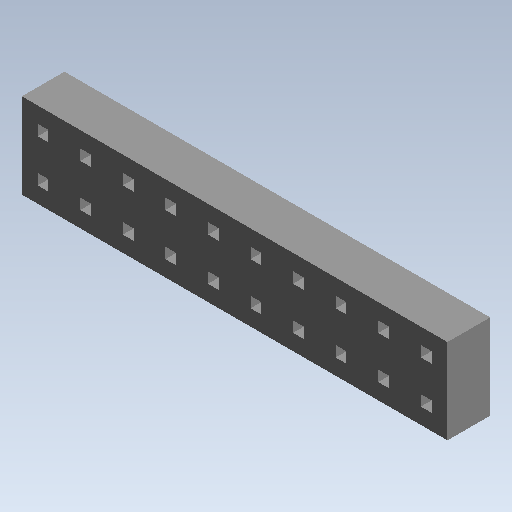
# Autodesk Inventor part: TB2TW-10-11-T-D-250-080
Saved by Autodesk Inventor 2021 (Build 250183000, 183)
## iProperties
Part Number: TB2TW-10-11-T-D-250-080
Material: Generic
Catalog Web Link: www.cadenas.de
Description: TW-TH Series Top Body-TW-TH Series
Vendor: SAMTEC
Document SubType Name: Modeling
Designer: partserver
Manufacturer: SAMTEC
Mass: 0.150089 g
Surface Area: 3.27452 cm^2
Volume: 0.150089 cm^3
Density: 1 g/cm^3
Appearance: PSOLRGB-175-175-175
Category: PARTsolutions
Company: SAMTEC
PSOL_IDENT_0: {$CADENAS_DATA\23d-libs\samtec\modelling\tw\parts\tw-th_top_body.prj},257 {VTYP=3D},{NB=TB2TW-10-11-
PSOL_IDENT_1: T-D-250-080},{LINA=TB2TW-10-11-T-D-250-080},{NN=TW-TH Series Top Body},{DATE=29.08.2019 09:17:19},{G
PSOL_IDENT_2: EOMDATE=10.06.2019 09:16:53},{VERSION=},{LINEID=10},{WBVAR=PINS,LEADST,PLOPT,ROWOPT,STACKERH,TAILL,P
PSOL_IDENT_3: OLARIZE},{WBNUMERIC=STACKERH}  {NB=TB2TW-10-11-T-D-250-080},{LINA=TB2TW-10-11-T-D-250-080},{KT=DUMMY
PSOL_IDENT_4: },{PN=TW-10-11-T-D-250-080},{SERIES=TW-TH},{PINS=10},{LEADST=11},{LEADSTALG=},{PLOPT=T},{PLOPTALG= '
PSOL_IDENT_5: -L','10micro\" (0,25 microm) Gold on contact, Matte Tin on tail','-S','30micro\" (0,76 microm) Gold
PSOL_IDENT_6: on contact, Matte Tin on tail' },{ROWOPT=D},{ROWOPTALG= '5','5:Five Row','6','6:Six Row','D','D:Doub
PSOL_IDENT_7: le Row','Q','Q:Quad Row','S','S:Single row','T','T:Triple Row' },{STACKERH=250},{STACKERHALG=[120:39
PSOL_IDENT_8: 7/5]},{TAILL=080},{TAILLALG='000','005','010','015','020','025','030','035','040','045','050','055','
PSOL_IDENT_9: 060','065','070','075','080','085','090','095','100','105','110','115','120','125','130','135','140'
PSOL_IDENT_10: ,'145'},{ALIGNMENTALG=x},{POLARIZE=Not Selected},{POLARIZEALG='001','002','003','004','005','006','0
PSOL_IDENT_11: 07','008','009','010','011','012','013','014','015','016','017','018','019','020'},{POLARIZEPN=},{KO
PSOL_IDENT_12: PTALG= '','Not Selected','-P','P:Plastic Pick and Place Pad' },{TROPTALG= '','Not Selected','-TR','T
PSOL_IDENT_13: R:Tape and Reel' },{IMAT=Black Liquid Crystal Polymer},{TM=Phosphor Bronze},{PLAT=Au or Sn over 50mi
PSOL_IDENT_14: cro\" (1,27 microm) Ni},{CR=5.2 A per pin (1 pin powered per row)},{OTEMP=-55°C to +125°C},{ROHSC=Ye
PSOL_IDENT_15: s},{L=0.7874},{W=0.1574},{OAL=0.397},{STACKERHMAX=397},{POLMAX='001','002','003','004','005','006','
PSOL_IDENT_16: 007','008','009','010','011','012','013','014','015','016','017','018','019','020','021','022','023'
PSOL_IDENT_17: ,'024','025','026','027','028','029','030','031','032','033','034','035','036','037','038','039','04
PSOL_IDENT_18: 0','041','042','043','044','045','046','047','048','049','050','051','052','053','054','055','056','
PSOL_IDENT_19: 057','058','059','060','061','062','063','064','065','066','067','068','069','070','071','072','073'
PSOL_IDENT_20: ,'074','075','076','077','078','079','080','081','082','083','084','085','086','087','088','089','09
PSOL_IDENT_21: 0','091','092','093','094','095','096','097','098','099','100','101','102','103','104','105','106','
PSOL_IDENT_22: 107','108','109','110','111','112','113','114','115','116','117','118','119','120','121','122','123'
PSOL_IDENT_23: ,'124','125','126','127','128','129','130','131','132','133','134','135','136','137','138','139','14
PSOL_IDENT_24: 0','141','142','143','144','145','146','147','148','149','150','151','152','153','154','155','156','
PSOL_IDENT_25: 157','158','159','160','161','162','163','164','165','166','167','168','169','170','171','172','173'
PSOL_IDENT_26: ,'174','175','176','177','178','179','180','181','182','183','184','185','186','187','188','189','19
PSOL_IDENT_27: 0','191','192','193','194','195','196','197','198','199','200','201','202','203','204','205','206','
PSOL_IDENT_28: 207','208','209','210','211','212','213','214','215','216','217','218','219','220','221','222','223'
PSOL_IDENT_29: ,'224','225','226','227','228','229','230','231','232','233','234','235','236','237','238','239','24
PSOL_IDENT_30: 0','241','242','243','244','245','246','247','248','249','250','251','252','253','254','255','256','
PSOL_IDENT_31: 257','258','259','260','261','262','263','264','265','266','267','268','269','270','271','272','273'
PSOL_IDENT_32: ,'274','275','276','277','278','279','280','281','282','283','284','285','286','287','288','289','29
PSOL_IDENT_33: 0','291','292','293','294','295','296','297','298','299','300'},{TEST2='001','002','003','004','005'
PSOL_IDENT_34: ,'006','007','008','009','010','011','012','013','014','015','016','017','018','019','020'},{TRUNC=2
PSOL_IDENT_35: 0},{MIN=0.147},{PINSNUM=10},{POLLR=0},{TAILLMAX=147},{TAILLRANGE='000','005','010','015','020','025'
PSOL_IDENT_36: ,'030','035','040','045','050','055','060','065','070','075','080','085','090','095','100','105','11
PSOL_IDENT_37: 0','115','120','125','130','135','140','145','150','155','160','165','170','175','180','185','190','
PSOL_IDENT_38: 195','200','205','210','215','220','225','230','235','240','245','250','255','260','265','270','275'
PSOL_IDENT_39: ,'280','285','290','295','300','305','310','315','320','325','330','335','340','345','350','355','36
PSOL_IDENT_40: 0','365','370','375','380','385','390','395','400','405','410','415','420','425','430','435','440','
PSOL_IDENT_41: 445','450','455','460','465','470','475','480','485','490','495','500','505','510','515','520','525'
PSOL_IDENT_42: ,'530','535','540','545','550','555','560','565','570','575','580','585','590','595','600','605','61
PSOL_IDENT_43: 0','615','620','625','630','635','640','645','650','655','660','665','670','675','680','685','690','
PSOL_IDENT_44: 695','700','705','710','715','720','725','730','735','740','745','750','755','760','765','770','775'
PSOL_IDENT_45: ,'780','785','790','795','800','805','810','815','820','825','830','835','840','845','850','855','86
PSOL_IDENT_46: 0','865','870','875','880','885','890','895','900','905','910','915','920','925','930','935','940','
PSOL_IDENT_47: 945','950','955','960','965','970','975','980','985','990','995'},{TAILLTRUNC=30},{TAILLNUM=0.08},{R
PSOL_IDENT_48: OWNO=2},{POLPLANEPOS=0},{POLPINPOS=0}
NB: TB2TW-10-11-T-D-250-080
NN: TW-TH Series Top Body
NT: TW-TH Series
NBSYN: TB2$PN.
LINA: TB2TW-10-11-T-D-250-080
CATALOG: Samtec
SERIES: TW-TH
PINS: 10
LEADST: 11
PLOPT: -T: Matte Tin Contact and Tail
ROWOPT: D:Double Row
STACKERH: 250
TAILL: 080
POLARIZE: Not Selected
IMAT: Black Liquid Crystal Polymer
TM: Phosphor Bronze
PLAT: Au or Sn over 50micro" (1,27 microm) Ni
CR: 5.2 A per pin (1 pin powered per row)
OTEMP: -55°C to +125°C
ROHSC: Yes
POLMAX: '001','002','003','004','005','006','007','008','009','010','011','012','013','014','015','016','017','018','019','020','021','022','023','024','025','026','027','028','029','030','031','032','033','034','035','036','037','038','039','040','041','042','043','044','045','046','047','048','049','050','051','052','053','054','055','056','057','058','059','060','061','062','063','064','065','066','067','068','069','070','071','072','073','074','075','076','077','078','079','080','081','082','083','084','085','086','087','088','089','090','091','092','093','094','095','096','097','098','099','100','101','102','103','104','105','106','107','108','109','110','111','112','113','114','115','116','117','118','119','120','121','122','123','124','125','126','127','128','129','130','131','132','133','134','135','136','137','138','139','140','141','142','143','144','145','146','147','148','149','150','151','152','153','154','155','156','157','158','159','160','161','162','163','164','165','166','167','168','169','170','171','172','173','174','175','176','177','178','179','180','181','182','183','184','185','186','187','188','189','190','191','192','193','194','195','196','197','198','199','200','201','202','203','204','205','206','207','208','209','210','211','212','213','214','215','216','217','218','219','220','221','222','223','224','225','226','227','228','229','230','231','232','233','234','235','236','237','238','239','240','241','242','243','244','245','246','247','248','249','250','251','252','253','254','255','256','257','258','259','260','261','262','263','264','265','266','267','268','269','270','271','272','273','274','275','276','277','278','279','280','281','282','283','284','285','286','287','288','289','290','291','292','293','294','295','296','297','298','299','300'
TAILLRANGE: '000','005','010','015','020','025','030','035','040','045','050','055','060','065','070','075','080','085','090','095','100','105','110','115','120','125','130','135','140','145','150','155','160','165','170','175','180','185','190','195','200','205','210','215','220','225','230','235','240','245','250','255','260','265','270','275','280','285','290','295','300','305','310','315','320','325','330','335','340','345','350','355','360','365','370','375','380','385','390','395','400','405','410','415','420','425','430','435','440','445','450','455','460','465','470','475','480','485','490','495','500','505','510','515','520','525','530','535','540','545','550','555','560','565','570','575','580','585','590','595','600','605','610','615','620','625','630','635','640','645','650','655','660','665','670','675','680','685','690','695','700','705','710','715','720','725','730','735','740','745','750','755','760','765','770','775','780','785','790','795','800','805','810','815','820','825','830','835','840','845','850','855','860','865','870','875','880','885','890','895','900','905','910','915','920','925','930','935','940','945','950','955','960','965','970','975','980','985','990','995'
SUPPLIER: SAMTEC
ARTICLENO: TB2TW-10-11-T-D-250-080
BOMINFO: TB2TW-10-11-T-D-250-080
CREATOR: CADENAS GmbH
Title: TB2TW-10-11-T-D-250-080
Author: Cadenas PARTsolutions
Comments: TW-TH Series
Autodesk Inventor part; units mm, degrees
ref_plane "YZ Plane" through (0, 0, 0) normal (1, 0, 0) x (0, 1, 0)
ref_plane "XZ Plane" through (0, 0, 0) normal (0, 1, 0) x (-1, 0, 0)
ref_plane "XY Plane" through (0, 0, 0) normal (0, 0, 1) x (1, 0, 0)
sketch "Sketch3" plane through (0, 6.35, 0) normal (0, 1, 0) x (-1, 0, 0)
  line L0 (-10, -1.999) -> (10, -1.999)
  line L1 (10, -1.999) -> (10, 1.999)
  line L2 (10, 1.999) -> (-10, 1.999)
  line L3 (-10, 1.999) -> (-10, -1.999)
  line L4 (8.746, 0.746) -> (9.254, 0.746)
  line L5 (9.254, 0.746) -> (9.254, 1.254)
  line L6 (9.254, 1.254) -> (8.746, 1.254)
  line L7 (8.746, 1.254) -> (8.746, 0.746)
  line L8 (8.746, -1.254) -> (9.254, -1.254)
  line L9 (9.254, -1.254) -> (9.254, -0.746)
  line L10 (9.254, -0.746) -> (8.746, -0.746)
  line L11 (8.746, -0.746) -> (8.746, -1.254)
  line L12 (6.746, 0.746) -> (7.254, 0.746)
  line L13 (7.254, 0.746) -> (7.254, 1.254)
  line L14 (7.254, 1.254) -> (6.746, 1.254)
  line L15 (6.746, 1.254) -> (6.746, 0.746)
  line L16 (6.746, -1.254) -> (7.254, -1.254)
  line L17 (7.254, -1.254) -> (7.254, -0.746)
  line L18 (7.254, -0.746) -> (6.746, -0.746)
  line L19 (6.746, -0.746) -> (6.746, -1.254)
  line L20 (4.746, 0.746) -> (5.254, 0.746)
  line L21 (5.254, 0.746) -> (5.254, 1.254)
  line L22 (5.254, 1.254) -> (4.746, 1.254)
  line L23 (4.746, 1.254) -> (4.746, 0.746)
  line L24 (4.746, -1.254) -> (5.254, -1.254)
  line L25 (5.254, -1.254) -> (5.254, -0.746)
  line L26 (5.254, -0.746) -> (4.746, -0.746)
  line L27 (4.746, -0.746) -> (4.746, -1.254)
  line L28 (2.746, 0.746) -> (3.254, 0.746)
  line L29 (3.254, 0.746) -> (3.254, 1.254)
  line L30 (3.254, 1.254) -> (2.746, 1.254)
  line L31 (2.746, 1.254) -> (2.746, 0.746)
  line L32 (2.746, -1.254) -> (3.254, -1.254)
  line L33 (3.254, -1.254) -> (3.254, -0.746)
  line L34 (3.254, -0.746) -> (2.746, -0.746)
  line L35 (2.746, -0.746) -> (2.746, -1.254)
  line L36 (0.746, 0.746) -> (1.254, 0.746)
  line L37 (1.254, 0.746) -> (1.254, 1.254)
  line L38 (1.254, 1.254) -> (0.746, 1.254)
  line L39 (0.746, 1.254) -> (0.746, 0.746)
  line L40 (0.746, -1.254) -> (1.254, -1.254)
  line L41 (1.254, -1.254) -> (1.254, -0.746)
  line L42 (1.254, -0.746) -> (0.746, -0.746)
  line L43 (0.746, -0.746) -> (0.746, -1.254)
  line L44 (-1.254, 0.746) -> (-0.746, 0.746)
  line L45 (-0.746, 0.746) -> (-0.746, 1.254)
  line L46 (-0.746, 1.254) -> (-1.254, 1.254)
  line L47 (-1.254, 1.254) -> (-1.254, 0.746)
  line L48 (-1.254, -1.254) -> (-0.746, -1.254)
  line L49 (-0.746, -1.254) -> (-0.746, -0.746)
  line L50 (-0.746, -0.746) -> (-1.254, -0.746)
  line L51 (-1.254, -0.746) -> (-1.254, -1.254)
  line L52 (-3.254, 0.746) -> (-2.746, 0.746)
  line L53 (-2.746, 0.746) -> (-2.746, 1.254)
  line L54 (-2.746, 1.254) -> (-3.254, 1.254)
  line L55 (-3.254, 1.254) -> (-3.254, 0.746)
  line L56 (-3.254, -1.254) -> (-2.746, -1.254)
  line L57 (-2.746, -1.254) -> (-2.746, -0.746)
  line L58 (-2.746, -0.746) -> (-3.254, -0.746)
  line L59 (-3.254, -0.746) -> (-3.254, -1.254)
  line L60 (-5.254, 0.746) -> (-4.746, 0.746)
  line L61 (-4.746, 0.746) -> (-4.746, 1.254)
  line L62 (-4.746, 1.254) -> (-5.254, 1.254)
  line L63 (-5.254, 1.254) -> (-5.254, 0.746)
  line L64 (-5.254, -1.254) -> (-4.746, -1.254)
  line L65 (-4.746, -1.254) -> (-4.746, -0.746)
  line L66 (-4.746, -0.746) -> (-5.254, -0.746)
  line L67 (-5.254, -0.746) -> (-5.254, -1.254)
  line L68 (-7.254, 0.746) -> (-6.746, 0.746)
  line L69 (-6.746, 0.746) -> (-6.746, 1.254)
  line L70 (-6.746, 1.254) -> (-7.254, 1.254)
  line L71 (-7.254, 1.254) -> (-7.254, 0.746)
  line L72 (-7.254, -1.254) -> (-6.746, -1.254)
  line L73 (-6.746, -1.254) -> (-6.746, -0.746)
  line L74 (-6.746, -0.746) -> (-7.254, -0.746)
  line L75 (-7.254, -0.746) -> (-7.254, -1.254)
  line L76 (-9.254, 0.746) -> (-8.746, 0.746)
  line L77 (-8.746, 0.746) -> (-8.746, 1.254)
  line L78 (-8.746, 1.254) -> (-9.254, 1.254)
  line L79 (-9.254, 1.254) -> (-9.254, 0.746)
  line L80 (-9.254, -1.254) -> (-8.746, -1.254)
  line L81 (-8.746, -1.254) -> (-8.746, -0.746)
  line L82 (-8.746, -0.746) -> (-9.254, -0.746)
  line L83 (-9.254, -0.746) -> (-9.254, -1.254)
  constraints: 168 end point
extrude "Extrusion1" add sketch "Sketch3" against normal blind 2.0066
ref_plane "0_XY" through (0, 0, 0) normal (0, 1, 0) x (1, 0, 0)
ref_plane "0_YZ" through (0, 0, 0) normal (1, 0, 0) x (0, 0, -1)
ref_plane "0_ZX" through (0, 0, 0) normal (0, 0, -1) x (0, 1, 0)
body "Solid1"
